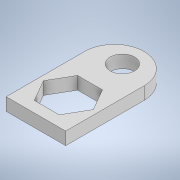
# Autodesk Inventor part: chapa
Saved by Autodesk Inventor 2021 (Build 250183000, 183)
## iProperties
Created: 2026-06-09
Part Number: chapa
Material: Generic
Document SubType Name: Sheet Metal
Designer: nelso
Density: 1 g/cm^3
Sheet Metal Rule: Default_mm
Appearance: Default
Author: nelso
Autodesk Inventor part; units mm, degrees
ref_plane "YZ Plane" through (0, 0, 0) normal (1, 0, 0) x (0, 1, 0)
ref_plane "XZ Plane" through (0, 0, 0) normal (0, 1, 0) x (-1, 0, 0)
ref_plane "XY Plane" through (0, 0, 0) normal (0, 0, 1) x (1, 0, 0)
sketch "Sketch1" plane through (0, 0, 0) normal (0, 1, 0) x (-1, 0, 0)
  line L0 (-11, 20) -> (11, 20)
  line L1 (11, 20) -> (11, -20)
  line L2 (11, -20) -> (-11, -20)
  line L3 (-11, -20) -> (-11, 20)
  line L4 (-11, 20) -> (11, -20) construction
  line L5 (11, 20) -> (-11, -20) construction
  line L6 (-11, -20) -> (-11, -12)
  line L7 (-11, 20) -> (-11, 9)
  line L8 (0, -20) -> (0, -12)
  line L9 (0, 20) -> (0, 8)
  line L10 (-4.6188, 0) -> (-9.2376, 8)
  line L11 (-9.2376, 8) -> (-4.6188, 16)
  line L12 (-4.6188, 16) -> (4.6188, 16)
  line L13 (4.6188, 16) -> (9.2376, 8)
  line L14 (9.2376, 8) -> (4.6188, 0)
  line L15 (4.6188, 0) -> (-4.6188, 0)
  dimension "d0" = 22
  dimension "d1" = 40
  dimension "d35" = 12
  dimension "d36" = 16
  constraints: 32 end point, 2 coincident, 2 midpoint, 2 parallel, 2 point on line, 2 vertical, 1 horizontal, 1 perpendicular, 13 other
  measures "d0" distance of L1.end L2.end
  measures "d1" distance of L0.end L1.end
  measures "d35" distance of L9.start L9.end
  measures "d36" distance between parallel lines of L12 L15
extrude "Plate1" add sketch "Sketch1" along normal blind 4.7 contours L0 L1 L2 L3 | L10 L11 L12 L13 L14 L15
hole "Hole4" at (0, 0, -12) direction (0, 1, 0) diameter 9 end through all clearance for "Countersunk Flat Head Screw ISO 2009/7046" size "M8" standard "ISO"
full round fillet "Fillet2" first side at (11, 1.5667, 6.6667) centre faces at (3.6667, 3.1333, -20) second side at (-11, 1.5667, -6.6667)
extrude "Cut1" cut sketch "Sketch1" along normal blind 4.7 contours L10 L11 L12 L13 L14 L15
equation "\"d31\" = Thickness"
equation "\"d37\" = Thickness"
equation "\"d3\" = Thickness"
equation "\"BendRadius\" = Thickness"
equation "\"BendReliefWidth\" = Thickness"
equation "\"BendReliefDepth\" = 0.5 * Thickness"
equation "\"CornerReliefSize\" = 4 * Thickness"
equation "\"MinimumRemnant\" = 2 * Thickness"
equation "\"TransitionRadius\" = BendRadius"
equation "\"JacobiRadiusSize\" = BendRadius"
equation "\"GapSize\" = Thickness"
equation "\"Thickness\" = 4.7"
body "Solid1"
